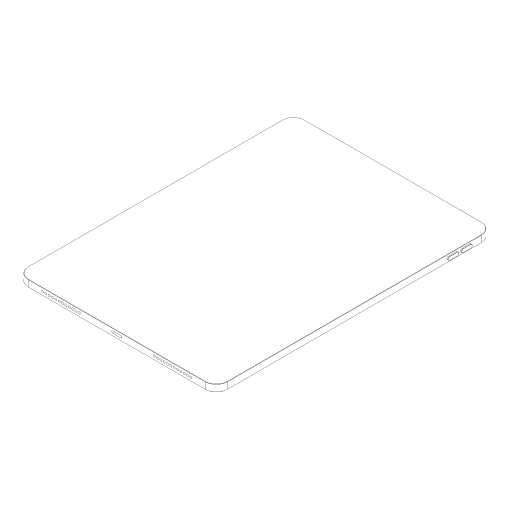
# Autodesk Inventor part: ipad
Saved by Autodesk Inventor 2024 (Build 280153000, 153)
## iProperties
Created: 2024-04-27
Part Number: ipad
Material: Generic
Document SubType Name: Modeling
Designer: alexz
Density: 1 g/cm^3
Appearance: Default
Author: alexz
Autodesk Inventor part; units mm, degrees
ref_plane "YZ Plane" through (0, 0, 0) normal (1, 0, 0) x (0, 1, 0)
ref_plane "XZ Plane" through (0, 0, 0) normal (0, 1, 0) x (-1, 0, 0)
ref_plane "XY Plane" through (0, 0, 0) normal (0, 0, 1) x (1, 0, 0)
sketch "Sketch1" plane through (0, 0, 0) normal (0, 1, 0) x (-1, 0, 0)
  line L0 (0, 0) -> (178.5, 0)
  line L1 (178.5, 0) -> (178.5, -247.6)
  line L2 (178.5, -247.6) -> (0, -247.6)
  line L3 (0, -247.6) -> (0, 0)
  dimension "d0" = 178.5
  dimension "d1" = 247.6
  constraints: 8 end point, 2 parallel, 1 horizontal, 1 perpendicular
  measures "d0" distance of L1.end L2.end
  measures "d1" distance of L0.end L1.end
extrude "Extrusion1" add sketch "Sketch1" along normal blind 6.1
fillet "Fillet1" radius 10 4 edges at (0, 3.05, 0) (0, 3.05, -247.6) (-178.5, 3.05, -247.6) (-178.5, 3.05, 0)
sketch "Sketch2" plane through (0, 0, -10) normal (1, 0, 0) x (0, 0, -1)
  line L0 (210.1, 3.05) -> (217.1, 3.05) construction
  line L1 (210.1, 1.55) -> (217.1, 1.55)
  line L2 (217.1, 4.55) -> (210.1, 4.55)
  arc A0 (210.1, 4.55) -> (210.1, 1.55) centre (210.1, 3.05) ccw
  arc A1 (217.1, 1.55) -> (217.1, 4.55) centre (217.1, 3.05) ccw
  line L3 (198.1, 3.05) -> (205.1, 3.05) construction
  line L4 (198.1, 1.55) -> (205.1, 1.55)
  line L5 (205.1, 4.55) -> (198.1, 4.55)
  arc A2 (198.1, 4.55) -> (198.1, 1.55) centre (198.1, 3.05) ccw
  arc A3 (205.1, 1.55) -> (205.1, 4.55) centre (205.1, 3.05) ccw
  line L6 (227.6, 6.1) -> (227.6, 0) projected
  point P0 (-10, 0)
  point P1 (213.6, 3.05)
  point P2 (218.6, 3.05)
  point P3 (208.6, 3.05)
  point P4 (201.6, 3.05)
  point P5 (206.6, 3.05)
  point P6 (196.6, 3.05)
  point P7 (227.6, 3.05)
  point P8 (227.6, 3.05)
  point P9 (227.6, 3.05)
  dimension "d5" = 7
  dimension "d6" = 3
  dimension "d8" = 7
  dimension "d9" = 3
  dimension "d10" = 2
  dimension "d11" = 9
  constraints: 16 end point, 12 point on circle, 8 tangent, 5 midpoint, 4 centre point, 2 horizontal, 2 horizontal alignment, 2 parallel
  measures "d5" distance of L0.start L0.end
  measures "d6" diameter of A1
  measures "d8" distance of L3.start L3.end
  measures "d9" diameter of A3
  measures "d10" distance of point (208.6, 3.05) point (206.6, 3.05)
  measures "d11" distance of point (227.6, 3.05) point (218.6, 3.05)
extrude "Extrusion2" add sketch "Sketch2" along normal blind 1
sketch "Sketch3" plane through (-10, 0, -247.6) normal (0, 0, -1) x (-1, 0, 0)
  line L0 (7, 3.05) -> (20, 3.05) construction
  line L1 (7, 1.05) -> (20, 1.05)
  line L2 (20, 5.05) -> (7, 5.05)
  arc A0 (7, 5.05) -> (7, 1.05) centre (7, 3.05) ccw
  arc A1 (20, 1.05) -> (20, 5.05) centre (20, 3.05) ccw
  line L3 (0, 0) -> (0, 6.1) projected
  circle A2 centre (28, 3.05) radius 1
  circle A3 centre (31, 3.05) radius 1
  circle A4 centre (34, 3.05) radius 1
  circle A5 centre (37, 3.05) radius 1
  circle A6 centre (40, 3.05) radius 1
  circle A7 centre (43, 3.05) radius 1
  circle A8 centre (46, 3.05) radius 1
  circle A9 centre (49, 3.05) radius 1
  circle A10 centre (52, 3.05) radius 1
  circle A11 centre (142.5, 3.05) radius 1
  circle A12 centre (139.5, 3.05) radius 1
  circle A13 centre (136.5, 3.05) radius 1
  circle A14 centre (133.5, 3.05) radius 1
  circle A15 centre (130.5, 3.05) radius 1
  circle A16 centre (127.5, 3.05) radius 1
  circle A17 centre (124.5, 3.05) radius 1
  circle A18 centre (121.5, 3.05) radius 1
  circle A19 centre (118.5, 3.05) radius 1
  line L4 (158.5, 6.1) -> (158.5, 0) projected
  line L5 (168.5, 0) -> (168.5, 6.1) projected
  circle A20 centre (115.5, 3.05) radius 1
  circle A21 centre (112.5, 3.05) radius 1
  circle A22 centre (109.5, 3.05) radius 1
  point P0 (-10, 0)
  point P1 (13.5, 3.05)
  point P2 (0, 3.05)
  point P3 (5, 3.05)
  point P4 (0, 3.05)
  point P5 (22, 3.05)
  point P6 (158.5, 3.05)
  dimension "d14" = 13
  dimension "d15" = 4
  dimension "d16" = 5
  dimension "d19" = 2
  dimension "d22" = 3
  dimension "d27" = 6
  dimension "d28" = 2
  dimension "d31" = 3
  dimension "d37" = 26
  dimension "d40" = 3
  constraints: 23 centre point, 8 end point, 6 point on circle, 4 horizontal, 4 midpoint, 4 tangent, 1 horizontal alignment, 1 parallel, 38 other
  measures "d14" distance of L0.start L0.end
  measures "d15" diameter of A1
  measures "d16" distance of point (0, 3.05) point (5, 3.05)
  measures "d19" diameter of A2
  measures "d22" distance of A2.centre A3.centre
  measures "d27" distance of A2.centre point (22, 3.05)
  measures "d28" diameter of A11
  measures "d31" distance of A11.centre A12.centre
  measures "d37" distance from line of L5 A11.centre
  measures "d40" distance of A19.centre A20.centre
extrude "Extrusion3" add sketch "Sketch3" along normal blind 1 contours A0 L2 A1 L1
extrude "Extrusion4" cut sketch "Sketch3" against normal blind 2 contours A2 | A3 | A4 | A5 | A6 | A7 | A8 | A9 | A10 | A11 | A12 | A13 | A14 | A15 | A16 | A17 | A18 | A19 | A20 | A21 | A22
sketch "Sketch4" plane through (-168.5, 0, 0) normal (0, 0, 1) x (1, 0, 0)
  line L0 (75.75, 3.1634) -> (82.75, 3.1634) construction
  line L1 (75.75, 2.1634) -> (82.75, 2.1634)
  line L2 (82.75, 4.1634) -> (75.75, 4.1634)
  arc A0 (75.75, 4.1634) -> (75.75, 2.1634) centre (75.75, 3.1634) ccw
  arc A1 (82.75, 2.1634) -> (82.75, 4.1634) centre (82.75, 3.1634) ccw
  line L3 (0, 6.1) -> (158.5, 6.1) projected
  circle A2 centre (112.75, 3.05) radius 1
  circle A3 centre (115.75, 3.05) radius 1
  circle A4 centre (118.75, 3.05) radius 1
  circle A5 centre (121.75, 3.05) radius 1
  circle A6 centre (124.75, 3.05) radius 1
  circle A7 centre (127.75, 3.05) radius 1
  circle A8 centre (130.75, 3.05) radius 1
  circle A9 centre (133.75, 3.05) radius 1
  circle A10 centre (136.75, 3.05) radius 1
  circle A11 centre (139.75, 3.05) radius 1
  circle A12 centre (142.75, 3.05) radius 1
  circle A13 centre (145.75, 3.05) radius 1
  circle A14 centre (45.75, 3.05) radius 1
  circle A15 centre (42.75, 3.05) radius 1
  circle A16 centre (39.75, 3.05) radius 1
  circle A17 centre (36.75, 3.05) radius 1
  circle A18 centre (33.75, 3.05) radius 1
  circle A19 centre (30.75, 3.05) radius 1
  circle A20 centre (27.75, 3.05) radius 1
  circle A21 centre (24.75, 3.05) radius 1
  circle A22 centre (21.75, 3.05) radius 1
  circle A23 centre (18.75, 3.05) radius 1
  circle A24 centre (15.75, 3.05) radius 1
  circle A25 centre (12.75, 3.05) radius 1
  point P0 (168.5, 0)
  point P1 (79.25, 3.1634)
  point P2 (79.25, 6.1)
  point P3 (83.75, 3.1634)
  point P4 (74.75, 3.1634)
  dimension "d47" = 7
  dimension "d48" = 2
  dimension "d49" = 2
  dimension "d50" = 29
  dimension "d53" = 3
  dimension "d58" = 2
  dimension "d59" = 29
  dimension "d62" = 3
  constraints: 26 centre point, 8 end point, 6 point on circle, 4 tangent, 3 horizontal, 2 midpoint, 1 parallel, 1 vertical alignment, 44 other
  measures "d47" distance of L0.start L0.end
  measures "d48" diameter of A1
  measures "d49" diameter of A2
  measures "d50" horizontal distance of point (83.75, 3.163) A2.centre
  measures "d53" distance of A2.centre A3.centre
  measures "d58" diameter of A14
  measures "d59" horizontal distance of A14.centre point (74.75, 3.163)
  measures "d62" distance of A14.centre A15.centre
extrude "Extrusion5" cut sketch "Sketch4" against normal blind 2 contours A2 | A3 | A4 | A5 | A6 | A7 | A8 | A9 | A10 | A11 | A12 | A13 | A14 | A15 | A16 | A17 | A18 | A19 | A20 | A21 | A22 | A23 | A24 | A25
extrude "Extrusion6" cut sketch "Sketch4" against normal blind 6 contours A0 L2 A1 L1
sketch "Sketch5" plane through (-168.5, 0, -6) normal (0, 0, 1) x (1, 0, 0)
  line L0 (75.75, 3.6634) -> (82.75, 3.6634)
  line L1 (82.75, 3.6634) -> (82.75, 2.6634)
  line L2 (82.75, 2.6634) -> (75.75, 2.6634)
  line L3 (75.75, 2.6634) -> (75.75, 3.6634)
  arc A0 (82.75, 2.1634) -> (82.75, 4.1634) centre (82.75, 3.1634) ccw projected
  line L4 (75.75, 4.1634) -> (82.75, 4.1634) projected
  point P0 (168.5, 0)
  point P1 (83.75, 3.1634)
  point P2 (82.75, 3.1634)
  point P3 (79.25, 4.1634)
  point P4 (79.25, 3.6634)
  dimension "d71" = 1
  constraints: 8 end point, 3 midpoint, 2 parallel, 1 horizontal, 1 horizontal alignment, 1 perpendicular, 1 point on circle, 1 vertical alignment
  measures "d71" distance of L0.end L1.end
extrude "Extrusion7" add sketch "Sketch5" along normal blind 4
fillet "Fillet2" radius 0.2 4 edges at (-92.75, 3.6634, -4) (-92.75, 2.6634, -4) (-85.75, 3.6634, -4) (-85.75, 2.6634, -4)
sketch "Sketch6" plane through (0, 0, 0) normal (0, -1, 0) x (1, 0, 0)
  circle A0 centre (-13, -234.6) radius 5
  circle A1 centre (-13, -234.6) radius 6
  line L0 (-10, -247.6) -> (-168.5, -247.6) projected
  line L1 (0, -10) -> (0, -237.6) projected
  point P0 (0, 0)
  dimension "d75" = 10
  dimension "d76" = 12
  dimension "d77" = 13
  dimension "d78" = 13
  constraints: 2 centre point, 1 coincident
  measures "d75" diameter of A0
  measures "d76" diameter of A1
  measures "d77" distance from line of L0 A0.centre
  measures "d78" distance from line of L1 A0.centre
extrude "Extrusion8" add sketch "Sketch6" along normal blind 2 contours A0 | A1
fillet "Fillet3" radius 1 1 edges at (-19, 0, -234.6)
fillet "Fillet4" radius 0.2 16 edges at (-2.9289, 6.1, -244.6711) (-89.25, 6.1, -247.6) (-175.5711, 6.1, -244.6711) (-178.5, 6.1, -123.8) (-175.5711, 6.1, -2.9289) (-89.25, 6.1, 0) (-2.9289, 6.1, -2.9289) (0, 6.1, -123.8) (-2.9289, 0, -244.6711) (-89.25, 0, -247.6) (-175.5711, 0, -244.6711) (-178.5, 0, -123.8) (-175.5711, 0, -2.9289) (-89.25, 0, 0) (-2.9289, 0, -2.9289) (0, 0, -123.8)
fillet "Fillet5" radius 0.1 12 edges at (1, 3.05, -206.6) (1, 1.55, -211.6) (1, 3.05, -216.6) (1, 4.55, -211.6) (1, 3.05, -218.6) (1, 1.55, -223.6) (1, 3.05, -228.6) (1, 4.55, -223.6) (-15, 3.05, -248.6) (-23.5, 1.05, -248.6) (-32, 3.05, -248.6) (-23.5, 5.05, -248.6)
body "Solid1"
